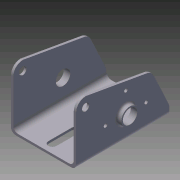
# Autodesk Inventor part: Ratchet Frame 1764
Saved by Autodesk Inventor 2011 (Build 150239000, 239)
## iProperties
Created: 2010-02-04
Part Number: Ratchet Frame 1764
Document SubType Name: Modeling
Designer: jrobinson
Density: 1 g/cm^3
Author: jrobinson
Autodesk Inventor part; units mm, degrees
ref_plane "YZ Plane" through (0, 0, 0) normal (1, 0, 0) x (0, 1, 0)
ref_plane "XZ Plane" through (0, 0, 0) normal (0, 1, 0) x (-1, 0, 0)
sketch "Sketch1" plane through (0, 0, 0) normal (0, 0, 1) x (1, 0, 0)
  line L0 (-26.1481, 3.048) -> (60.2119, 3.048)
  line L1 (60.2119, 3.048) -> (60.2119, 0)
  line L2 (60.2119, 0) -> (-26.1481, 0)
  line L3 (-26.1481, 0) -> (-26.1481, 3.048)
  line L4 (-26.1481, 0) -> (-23.1001, 0)
  line L5 (-23.1001, 0) -> (-23.1001, 78.613)
  line L6 (-23.1001, 78.613) -> (-26.1481, 78.613)
  line L7 (-26.1481, 78.613) -> (-26.1481, 0)
  line L8 (60.2119, 0) -> (57.1639, 0)
  line L9 (57.1639, 0) -> (57.1639, 78.613)
  line L10 (57.1639, 78.613) -> (60.2119, 78.613)
  line L11 (60.2119, 78.613) -> (60.2119, 0)
  point P0 (0, 0)
  dimension "d0" = 86.36
  dimension "d1" = 3.048
  dimension "d2" = 3.048
  dimension "d3" = 3.048
  dimension "d4" = 78.613
  dimension "d5" = 0
  constraints: 24 end point, 6 parallel, 3 horizontal, 3 perpendicular
  measures "d0" distance of L1.end L2.end
  measures "d1" distance between parallel lines of L7 L5
  measures "d2" distance between parallel lines of L0 L2
  measures "d3" distance between parallel lines of L11 L9
  measures "d4" distance between parallel lines of L2 L6
  measures "d5" distance from line of L5.end L10
extrude "Extrusion1" add sketch "Sketch1" along normal blind 123.7488
fillet "Fillet1" radius 12.7 2 edges at (58.6879, 78.613, 123.7488) (-24.6241, 78.613, 123.7488)
sketch "Sketch2" plane through (60.2119, 0, 0) normal (1, 0, 0) x (0, 0, -1)
  arc A0 (-111.0488, 78.613) -> (-123.7488, 65.913) centre (-111.0488, 65.913) ccw projected
  circle A1 centre (-111.0488, 65.913) radius 4.7625
  dimension "d9" = 9.525
  constraints: 1 centre point, 1 coincident
  measures "d9" diameter of A1
extrude "Extrusion2" cut sketch "Sketch2" against normal through all
fillet "Fillet2" radius 6.35 4 edges at (57.1639, 3.048, 61.8744) (60.2119, 0, 61.8744) (-23.1001, 3.048, 61.8744) (-26.1481, 0, 61.8744)
sketch "Sketch3" plane through (60.2119, 78.613, 111.0488) normal (1, 0, 0) x (0, 0, -1)
  line L0 (111.0488, -72.263) -> (-12.7, -72.263) projected
  line L1 (111.0488, -72.263) -> (111.0488, 0) projected
  line L2 (111.0488, 0) -> (0, 0) projected
  line L3 (-12.7, -12.7) -> (-12.7, -72.263) projected
  line L4 (111.0488, -65.913) -> (-12.7, -65.913)
  line L5 (0, 0) -> (87.5082, -15.4301)
  line L6 (87.5082, -15.4301) -> (111.0488, -65.913)
  point P0 (111.0488, -78.613)
  dimension "d13" = 6.35
  dimension "d15" = 125
  dimension "d16" = 65
  constraints: 6 end point, 2 point on line, 1 perpendicular
  measures "d13" distance between parallel lines of L0 L4
  measures "d15" angle of L6 L5
  measures "d16" angle of L6 L4
extrude "Extrusion3" cut sketch "Sketch3" against normal through all contours L6 L5 L2 L1
fillet "Fillet3" radius 12.7 2 edges at (58.6879, 63.1829, 23.5406) (-24.6241, 63.1829, 23.5406)
fillet "Fillet4" radius 12.7 2 edges at (58.6879, 12.7, 0) (-24.6241, 12.7, 0)
sketch "Sketch4" plane through (-16.7501, 3.048, 0) normal (0, 1, 0) x (1, 0, 0)
  line L0 (0, -123.7488) -> (67.564, -123.7488) projected
  line L1 (67.564, 0) -> (0, 0) projected
  circle A0 centre (33.782, -11.7475) radius 5.3975
  circle A1 centre (33.782, -37.1475) radius 5.3975
  arc A2 (28.3845, -112.002) -> (39.1795, -112.002) centre (33.782, -112.0013) ccw
  arc A3 (39.1833, -81.0902) -> (28.3807, -81.0902) centre (33.782, -81.0895) ccw
  line L2 (28.3845, -112.002) -> (28.3807, -81.0902)
  line L3 (39.1833, -81.0902) -> (39.1795, -112.002)
  point P0 (16.7501, 0)
  dimension "d21" = 10.795
  dimension "d22" = 10.795
  dimension "d23" = 25.4
  dimension "d24" = 11.7475
  dimension "d25" = 10.795
  dimension "d26" = 10.8026
  dimension "d27" = 11.7475
  dimension "d28" = 30.9118
  dimension "d29" = 30.9118
  dimension "d30" = 30.9118
  constraints: 4 centre point, 4 end point, 4 point on circle, 3 tangent
  measures "d21" diameter of A0
  measures "d22" diameter of A1
  measures "d23" distance of A0.centre A1.centre
  measures "d24" distance from line of L1 A0.centre
  measures "d25" diameter of A2
  measures "d26" diameter of A3
  measures "d27" distance from line of L0 A2.centre
  measures "d28" distance of A2.centre A3.centre
  measures "d29" distance of L2.start L2.end
  measures "d30" distance of L3.start L3.end
extrude "Extrusion4" cut sketch "Sketch4" against normal through all
sketch "Sketch5" plane through (60.2119, 6.35, 123.7488) normal (1, 0, 0) x (0, 0, -1)
  circle A0 centre (12.7, 59.563) radius 4.7625 projected
  circle A1 centre (66.064, 25.146) radius 9.525
  circle A2 centre (66.064, 25.146) radius 11.43
  line L0 (0, -6.35) -> (123.7488, -6.35) projected
  dimension "d33" = 19.05
  dimension "d36" = 22.86
  dimension "d37" = 31.496
  dimension "d38" = 63.5
  constraints: 2 centre point, 1 coincident
  measures "d33" diameter of A1
  measures "d36" diameter of A2
  measures "d37" distance from line of A1.centre L0
  measures "d38" distance of A1.centre A0.centre
extrude "Extrusion5" add sketch "Sketch5" along normal blind 5.461 contours A2
sketch "Sketch6" plane through (60.2119, 31.496, 57.6848) normal (1, 0, 0) x (0, 0, -1)
  circle A0 centre (0, 0) radius 9.525 projected
  point P0 (57.6848, -31.496)
ref_plane "Work Plane1" through (17.0319, 0, 117.3988) normal (1, 0, 0) x (0, 1, 0)
mirror "Mirror1" about plane through (17.0319, 0, 117.3988) normal (1, 0, 0) of "Extrusion5"
extrude "Extrusion6" cut sketch "Sketch6" against normal through all
fillet "Fillet5" radius 2.54 2 edges at (60.2119, 31.496, 69.1148) (-26.1482, 31.496, 69.1148)
sketch "Sketch7" plane through (60.2119, 6.35, 123.7488) normal (1, 0, 0) x (0, 0, -1)
  circle A0 centre (39.0765, 25.1459) radius 2.317 projected
  circle A1 centre (93.0515, 25.1461) radius 2.317 projected
  circle A2 centre (66.064, 25.146) radius 14.2875 projected
  line L0 (97.8141, -6.6039) -> (97.814, 56.8961) projected
  line L1 (34.3141, -6.6041) -> (97.8141, -6.6039) projected
  line L2 (34.314, 56.8959) -> (34.3141, -6.6041) projected
  line L3 (97.814, 56.8961) -> (34.314, 56.8959) projected
  circle A3 centre (66.0641, -1.8415) radius 2.317 projected
  circle A4 centre (66.064, 52.1335) radius 2.317 projected
  point P0 (123.7488, -6.35)
extrude "Extrusion7" cut sketch "Sketch7" against normal up to surface (3.048 mm away) contours A0 | A1 | A4
equation "\"d27\" = d24"
equation "\"d29\" = d28"
body "Solid1"
